Autodesk Inventor part; units mm, degrees
(part 3 of 3)
sketch "Sketch3" plane through (0, 0, 0) normal (0, -1, 0) x (1, 0, 0)
  line L0 (7.891, 22.7422) -> (7.891, -2.8235) construction
  line L1 (7.891, -2.8235) -> (4.151, -2.8235) construction
  line L2 (4.151, -2.8235) -> (4.151, 22.7422) construction
  line L3 (4.151, 22.7422) -> (7.891, 22.7422) construction
  line L4 (5.4758, -4.9863) -> (5.4758, -20.3165) construction
  line L5 (5.4758, -20.3165) -> (-4.0194, -20.3165) construction
  line L6 (-4.0194, -20.3165) -> (-4.0194, -4.9863) construction
  line L7 (-4.0194, -4.9863) -> (5.4758, -4.9863) construction
  line L8 (4.2338, 13.0137) -> (4.2338, 14.1137)
  line L9 (4.2338, 14.1137) -> (5.5167, 15.068)
  line L10 (5.5167, 15.068) -> (5.5167, 15.488)
  line L11 (5.5167, 15.488) -> (4.2338, 15.488)
  line L12 (4.2338, 15.488) -> (4.2338, 16.3851)
  line L13 (4.2338, 16.3851) -> (7.7338, 16.3851)
  line L14 (7.7338, 16.3851) -> (7.7338, 14.8708)
  spline S0 degree 2 poles (7.7338, 14.8708) (7.7338, 14.5594) (7.6624, 14.1137) (7.5453, 13.9194) knots 0 0 0 1 2 2 2
  spline S1 degree 2 poles (7.5453, 13.9194) (7.4281, 13.7194) (7.0538, 13.488) (6.771, 13.488) knots 0 0 0 1 2 2 2
  spline S2 degree 2 poles (6.771, 13.488) (6.3853, 13.488) (5.8938, 13.848) (5.7338, 14.1822) knots 0 0 0 1 2 2 2
  line L15 (5.7338, 14.1822) -> (4.2338, 13.0137)
  spline S3 degree 2 poles (6.6624, 14.4222) (6.7938, 14.4222) (6.9824, 14.5308) (7.0367, 14.6622) knots 0 0 0 1 2 2 2
  spline S4 degree 2 poles (7.0367, 14.6622) (7.0738, 14.7537) (7.091, 14.9994) (7.091, 15.1622) knots 0 0 0 1 2 2 2
  line L16 (7.091, 15.1622) -> (7.091, 15.488)
  line L17 (7.091, 15.488) -> (6.1481, 15.488)
  line L18 (6.1481, 15.488) -> (6.1481, 15.2108)
  spline S5 degree 2 poles (6.1481, 15.2108) (6.1481, 14.9937) (6.191, 14.7022) (6.2653, 14.6022) knots 0 0 0 1 2 2 2
  spline S6 degree 2 poles (6.2653, 14.6022) (6.3395, 14.508) (6.5138, 14.4222) (6.6624, 14.4222) knots 0 0 0 1 2 2 2
  spline S7 degree 2 poles (5.5538, 9.9651) (4.9024, 9.9651) (4.151, 10.7251) (4.151, 11.4108) knots 0 0 0 1 2 2 2
  spline S8 degree 2 poles (4.151, 11.4108) (4.151, 12.0994) (4.9024, 12.8594) (5.5538, 12.8594) knots 0 0 0 1 2 2 2
  spline S9 degree 2 poles (5.5538, 12.8594) (6.2081, 12.8594) (6.9567, 12.0937) (6.9567, 11.4108) knots 0 0 0 1 2 2 2
  spline S10 degree 2 poles (6.9567, 11.4108) (6.9567, 10.7194) (6.2053, 9.9651) (5.5538, 9.9651) knots 0 0 0 1 2 2 2
  spline S11 degree 2 poles (4.911, 11.008) (5.0138, 10.9251) (5.2967, 10.8422) (5.5481, 10.8422) knots 0 0 0 1 2 2 2
  spline S12 degree 2 poles (5.5481, 10.8422) (5.7795, 10.8422) (6.0938, 10.928) (6.1881, 11.0022) knots 0 0 0 1 2 2 2
  spline S13 degree 2 poles (6.1881, 11.0022) (6.2853, 11.0765) (6.3653, 11.2908) (6.3653, 11.4108) knots 0 0 0 1 2 2 2
  spline S14 degree 2 poles (6.3653, 11.4108) (6.3653, 11.5337) (6.2995, 11.7251) (6.1995, 11.8137) knots 0 0 0 1 2 2 2
  spline S15 degree 2 poles (6.1995, 11.8137) (6.1081, 11.8908) (5.791, 11.9822) (5.5481, 11.9822) knots 0 0 0 1 2 2 2
  spline S16 degree 2 poles (5.5481, 11.9822) (5.331, 11.9822) (5.0138, 11.9022) (4.9195, 11.8251) knots 0 0 0 1 2 2 2
  spline S17 degree 2 poles (4.9195, 11.8251) (4.8281, 11.748) (4.7424, 11.5394) (4.7424, 11.4051) knots 0 0 0 1 2 2 2
  spline S18 degree 2 poles (4.7424, 11.4051) (4.7424, 11.2908) (4.8195, 11.0794) (4.911, 11.008) knots 0 0 0 1 2 2 2
  spline S19 degree 2 poles (5.591, 6.6051) (4.9681, 6.6051) (4.1824, 7.2937) (4.1824, 7.808) knots 0 0 0 1 2 2 2
  spline S20 degree 2 poles (4.1824, 7.808) (4.1824, 8.028) (4.2767, 8.3594) (4.3653, 8.5108) knots 0 0 0 1 2 2 2
  line L19 (4.3653, 8.5108) -> (4.2338, 8.5451)
  line L20 (4.2338, 8.5451) -> (4.2338, 9.3594)
  line L21 (4.2338, 9.3594) -> (7.891, 9.3594)
  line L22 (7.891, 9.3594) -> (7.891, 8.5108)
  line L23 (7.891, 8.5108) -> (6.5967, 8.5108)
  spline S21 degree 2 poles (6.5967, 8.5108) (6.7538, 8.3165) (6.9453, 7.9108) (6.9453, 7.6451) knots 0 0 0 1 2 2 2
  spline S22 degree 2 poles (6.9453, 7.6451) (6.9453, 7.1451) (6.2253, 6.6051) (5.591, 6.6051) knots 0 0 0 1 2 2 2
  spline S23 degree 2 poles (5.571, 7.4765) (5.9224, 7.4765) (6.3024, 7.7165) (6.3024, 8.0222) knots 0 0 0 1 2 2 2
  spline S24 degree 2 poles (6.3024, 8.0222) (6.3024, 8.1422) (6.231, 8.3965) (6.1624, 8.5108) knots 0 0 0 1 2 2 2
  line L24 (6.1624, 8.5108) -> (4.8424, 8.5108)
  spline S25 degree 2 poles (4.8424, 8.5108) (4.8081, 8.4194) (4.7853, 8.2565) (4.7853, 8.1394) knots 0 0 0 1 2 2 2
  spline S26 degree 2 poles (4.7853, 8.1394) (4.7853, 7.8051) (5.1795, 7.4765) (5.571, 7.4765) knots 0 0 0 1 2 2 2
  spline S27 degree 2 poles (5.5538, 3.2937) (4.9024, 3.2937) (4.151, 4.0537) (4.151, 4.7394) knots 0 0 0 1 2 2 2
  spline S28 degree 2 poles (4.151, 4.7394) (4.151, 5.428) (4.9024, 6.188) (5.5538, 6.188) knots 0 0 0 1 2 2 2
  spline S29 degree 2 poles (5.5538, 6.188) (6.2081, 6.188) (6.9567, 5.4222) (6.9567, 4.7394) knots 0 0 0 1 2 2 2
  spline S30 degree 2 poles (6.9567, 4.7394) (6.9567, 4.048) (6.2053, 3.2937) (5.5538, 3.2937) knots 0 0 0 1 2 2 2
  spline S31 degree 2 poles (4.911, 4.3365) (5.0138, 4.2537) (5.2967, 4.1708) (5.5481, 4.1708) knots 0 0 0 1 2 2 2
  spline S32 degree 2 poles (5.5481, 4.1708) (5.7795, 4.1708) (6.0938, 4.2565) (6.1881, 4.3308) knots 0 0 0 1 2 2 2
  spline S33 degree 2 poles (6.1881, 4.3308) (6.2853, 4.4051) (6.3653, 4.6194) (6.3653, 4.7394) knots 0 0 0 1 2 2 2
  spline S34 degree 2 poles (6.3653, 4.7394) (6.3653, 4.8622) (6.2995, 5.0537) (6.1995, 5.1422) knots 0 0 0 1 2 2 2
  spline S35 degree 2 poles (6.1995, 5.1422) (6.1081, 5.2194) (5.791, 5.3108) (5.5481, 5.3108) knots 0 0 0 1 2 2 2
  spline S36 degree 2 poles (5.5481, 5.3108) (5.331, 5.3108) (5.0138, 5.2308) (4.9195, 5.1537) knots 0 0 0 1 2 2 2
  spline S37 degree 2 poles (4.9195, 5.1537) (4.8281, 5.0765) (4.7424, 4.868) (4.7424, 4.7337) knots 0 0 0 1 2 2 2
  spline S38 degree 2 poles (4.7424, 4.7337) (4.7424, 4.6194) (4.8195, 4.408) (4.911, 4.3365) knots 0 0 0 1 2 2 2
  spline S39 degree 2 poles (-0.5256, 12.428) (-0.7799, 12.428) (-1.1799, 12.6337) (-1.3113, 12.8108) knots 0 0 0 1 2 2 2
  spline S40 degree 2 poles (-1.3113, 12.8108) (-1.4656, 13.0194) (-1.5971, 13.5137) (-1.5971, 13.8965) knots 0 0 0 1 2 2 2
  line L25 (-1.5971, 13.8965) -> (-1.5971, 15.4251)
  line L26 (-1.5971, 15.4251) -> (1.9029, 15.4251)
  line L27 (1.9029, 15.4251) -> (1.9029, 14.0651)
  spline S41 degree 2 poles (1.9029, 14.0651) (1.9029, 13.6422) (1.8458, 13.2508) (1.7515, 13.0565) knots 0 0 0 1 2 2 2
  spline S42 degree 2 poles (1.7515, 13.0565) (1.6487, 12.8565) (1.3087, 12.6622) (1.0887, 12.6622) knots 0 0 0 1 2 2 2
  spline S43 degree 2 poles (1.0887, 12.6622) (0.8344, 12.6622) (0.4487, 12.9308) (0.3401, 13.1765) knots 0 0 0 1 2 2 2
  line L28 (0.3401, 13.1765) -> (0.3201, 13.1765)
  spline S44 degree 2 poles (0.3201, 13.1765) (0.2515, 12.8308) (-0.1742, 12.428) (-0.5256, 12.428) knots 0 0 0 1 2 2 2
  spline S45 degree 2 poles (-0.5113, 13.3651) (-0.3428, 13.3651) (-0.1628, 13.4937) (-0.1171, 13.6508) knots 0 0 0 1 2 2 2
  spline S46 degree 2 poles (-0.1171, 13.6508) (-0.0885, 13.7565) (-0.0828, 14.128) (-0.0828, 14.3308) knots 0 0 0 1 2 2 2
  line L29 (-0.0828, 14.3308) -> (-0.0828, 14.528)
  line L30 (-0.0828, 14.528) -> (-0.9542, 14.528)
  line L31 (-0.9542, 14.528) -> (-0.9542, 14.4622)
  spline S47 degree 2 poles (-0.9542, 14.4622) (-0.9542, 14.0794) (-0.9485, 13.7508) (-0.8913, 13.6137) knots 0 0 0 1 2 2 2
  spline S48 degree 2 poles (-0.8913, 13.6137) (-0.8313, 13.4708) (-0.6371, 13.3651) (-0.5113, 13.3651) knots 0 0 0 1 2 2 2
  spline S49 degree 2 poles (0.9115, 13.5851) (1.0001, 13.5851) (1.1744, 13.6737) (1.2144, 13.7822) knots 0 0 0 1 2 2 2
  spline S50 degree 2 poles (1.2144, 13.7822) (1.2544, 13.8822) (1.2601, 14.1765) (1.2601, 14.4422) knots 0 0 0 1 2 2 2
  line L32 (1.2601, 14.4422) -> (1.2601, 14.528)
  line L33 (1.2601, 14.528) -> (0.5201, 14.528)
  line L34 (0.5201, 14.528) -> (0.5201, 14.3851)
  spline S51 degree 2 poles (0.5201, 14.3851) (0.5201, 14.1708) (0.5344, 13.8708) (0.5744, 13.7822) knots 0 0 0 1 2 2 2
  spline S52 degree 2 poles (0.5744, 13.7822) (0.6287, 13.6594) (0.8001, 13.5851) (0.9115, 13.5851) knots 0 0 0 1 2 2 2
  line L35 (0.2372, 9.888) -> (0.2372, 9.9622)
  spline S53 degree 2 poles (0.2372, 9.9622) (0.2572, 10.0165) (0.2744, 10.2565) (0.2744, 10.3365) knots 0 0 0 1 2 2 2
  spline S54 degree 2 poles (0.2744, 10.3365) (0.2744, 10.5165) (0.2287, 10.7937) (0.1715, 10.9537) knots 0 0 0 1 2 2 2
  line L36 (0.1715, 10.9537) -> (-1.5971, 10.9537)
  line L37 (-1.5971, 10.9537) -> (-1.5971, 11.8022)
  line L38 (-1.5971, 11.8022) -> (1.0429, 11.8022)
  line L39 (1.0429, 11.8022) -> (1.0429, 10.9537)
  line L40 (1.0429, 10.9537) -> (0.6544, 10.9537)
  spline S55 degree 2 poles (0.6544, 10.9537) (0.8944, 10.6737) (1.0515, 10.2622) (1.0515, 10.088) knots 0 0 0 1 2 2 2
  spline S56 degree 2 poles (1.0515, 10.088) (1.0515, 10.0422) (1.0458, 9.9308) (1.0429, 9.888) knots 0 0 0 1 2 2 2
  line L41 (1.0429, 9.888) -> (0.2372, 9.888)
  line L42 (0.2372, 7.4937) -> (0.2372, 7.568)
  spline S57 degree 2 poles (0.2372, 7.568) (0.2572, 7.6222) (0.2744, 7.8622) (0.2744, 7.9422) knots 0 0 0 1 2 2 2
  spline S58 degree 2 poles (0.2744, 7.9422) (0.2744, 8.1222) (0.2287, 8.3994) (0.1715, 8.5594) knots 0 0 0 1 2 2 2
  line L43 (0.1715, 8.5594) -> (-1.5971, 8.5594)
  line L44 (-1.5971, 8.5594) -> (-1.5971, 9.408)
  line L45 (-1.5971, 9.408) -> (1.0429, 9.408)
  line L46 (1.0429, 9.408) -> (1.0429, 8.5594)
  line L47 (1.0429, 8.5594) -> (0.6544, 8.5594)
  spline S59 degree 2 poles (0.6544, 8.5594) (0.8944, 8.2794) (1.0515, 7.868) (1.0515, 7.6937) knots 0 0 0 1 2 2 2
  spline S60 degree 2 poles (1.0515, 7.6937) (1.0515, 7.648) (1.0458, 7.5365) (1.0429, 7.4937) knots 0 0 0 1 2 2 2
  line L48 (1.0429, 7.4937) -> (0.2372, 7.4937)
  line L49 (-1.5971, 4.448) -> (-1.5971, 5.2965)
  line L50 (-1.5971, 5.2965) -> (-1.3228, 5.2965)
  spline S61 degree 2 poles (-1.3228, 5.2965) (-1.4999, 5.5137) (-1.6713, 5.8937) (-1.6713, 6.1451) knots 0 0 0 1 2 2 2
  spline S62 degree 2 poles (-1.6713, 6.1451) (-1.6713, 6.6251) (-0.9285, 7.2022) (-0.2971, 7.2022) knots 0 0 0 1 2 2 2
  spline S63 degree 2 poles (-0.2971, 7.2022) (0.0372, 7.2022) (0.5572, 7.008) (0.7429, 6.8394) knots 0 0 0 1 2 2 2
  spline S64 degree 2 poles (0.7429, 6.8394) (0.9201, 6.6794) (1.1144, 6.2222) (1.1144, 5.9965) knots 0 0 0 1 2 2 2
  spline S65 degree 2 poles (1.1144, 5.9965) (1.1144, 5.7594) (1.0144, 5.4565) (0.9344, 5.2965) knots 0 0 0 1 2 2 2
  line L51 (0.9344, 5.2965) -> (2.0601, 5.2965)
  line L52 (2.0601, 5.2965) -> (2.0601, 4.448)
  line L53 (2.0601, 4.448) -> (-1.5971, 4.448)
  line L54 (-0.8713, 5.2965) -> (0.4258, 5.2965)
  spline S66 degree 2 poles (0.4258, 5.2965) (0.4629, 5.3851) (0.4972, 5.5822) (0.4972, 5.6651) knots 0 0 0 1 2 2 2
  spline S67 degree 2 poles (0.4972, 5.6651) (0.4972, 5.9965) (0.0801, 6.3308) (-0.2885, 6.3308) knots 0 0 0 1 2 2 2
  spline S68 degree 2 poles (-0.2885, 6.3308) (-0.6771, 6.3308) (-1.0285, 6.0622) (-1.0285, 5.768) knots 0 0 0 1 2 2 2
  spline S69 degree 2 poles (-1.0285, 5.768) (-1.0285, 5.6537) (-0.9428, 5.3937) (-0.8713, 5.2965) knots 0 0 0 1 2 2 2
  line L55 (-7.4279, 15.1337) -> (-7.4279, 16.0137)
  line L56 (-7.4279, 16.0137) -> (-6.5051, 16.0137)
  line L57 (-6.5051, 16.0137) -> (-6.5051, 15.1337)
  line L58 (-6.5051, 15.1337) -> (-7.4279, 15.1337)
  spline S70 degree 2 poles (-7.4994, 12.9308) (-7.4994, 13.2765) (-7.3336, 13.848) (-7.1622, 14.0594) knots 0 0 0 1 2 2 2
  spline S71 degree 2 poles (-7.1622, 14.0594) (-6.9908, 14.268) (-6.4708, 14.4994) (-6.1194, 14.4994) knots 0 0 0 1 2 2 2
  spline S72 degree 2 poles (-6.1194, 14.4994) (-5.7508, 14.4994) (-5.2136, 14.2537) (-5.0394, 14.0308) knots 0 0 0 1 2 2 2
  spline S73 degree 2 poles (-5.0394, 14.0308) (-4.8708, 13.8165) (-4.7165, 13.2594) (-4.7165, 12.9565) knots 0 0 0 1 2 2 2
  spline S74 degree 2 poles (-4.7165, 12.9565) (-4.7165, 12.688) (-4.8336, 12.2308) (-4.9279, 12.0337) knots 0 0 0 1 2 2 2
  line L59 (-4.9279, 12.0337) -> (-5.6508, 12.0337)
  line L60 (-5.6508, 12.0337) -> (-5.6508, 12.1537)
  spline S75 degree 2 poles (-5.6508, 12.1537) (-5.6079, 12.2022) (-5.4936, 12.3422) (-5.4394, 12.4422) knots 0 0 0 1 2 2 2
  spline S76 degree 2 poles (-5.4394, 12.4422) (-5.3879, 12.5394) (-5.3194, 12.768) (-5.3194, 12.9194) knots 0 0 0 1 2 2 2
  spline S77 degree 2 poles (-5.3194, 12.9194) (-5.3194, 13.2594) (-5.7508, 13.6222) (-6.1194, 13.6222) knots 0 0 0 1 2 2 2
  spline S78 degree 2 poles (-6.1194, 13.6222) (-6.5022, 13.6222) (-6.8965, 13.248) (-6.8965, 12.908) knots 0 0 0 1 2 2 2
  spline S79 degree 2 poles (-6.8965, 12.908) (-6.8965, 12.748) (-6.8222, 12.4908) (-6.7736, 12.408) knots 0 0 0 1 2 2 2
  spline S80 degree 2 poles (-6.7736, 12.408) (-6.7279, 12.328) (-6.6222, 12.2051) (-6.5736, 12.1537) knots 0 0 0 1 2 2 2
  line L61 (-6.5736, 12.1537) -> (-6.5736, 12.0337)
  line L62 (-6.5736, 12.0337) -> (-7.2936, 12.0337)
  spline S81 degree 2 poles (-7.2936, 12.0337) (-7.3879, 12.2337) (-7.4994, 12.668) (-7.4994, 12.9308) knots 0 0 0 1 2 2 2
  spline S82 degree 2 poles (-6.1079, 8.7737) (-6.7594, 8.7737) (-7.5108, 9.5337) (-7.5108, 10.2194) knots 0 0 0 1 2 2 2
  spline S83 degree 2 poles (-7.5108, 10.2194) (-7.5108, 10.908) (-6.7594, 11.668) (-6.1079, 11.668) knots 0 0 0 1 2 2 2
  spline S84 degree 2 poles (-6.1079, 11.668) (-5.4536, 11.668) (-4.7051, 10.9022) (-4.7051, 10.2194) knots 0 0 0 1 2 2 2
  spline S85 degree 2 poles (-4.7051, 10.2194) (-4.7051, 9.528) (-5.4565, 8.7737) (-6.1079, 8.7737) knots 0 0 0 1 2 2 2
  spline S86 degree 2 poles (-6.7508, 9.8165) (-6.6479, 9.7337) (-6.3651, 9.6508) (-6.1136, 9.6508) knots 0 0 0 1 2 2 2
  spline S87 degree 2 poles (-6.1136, 9.6508) (-5.8822, 9.6508) (-5.5679, 9.7365) (-5.4736, 9.8108) knots 0 0 0 1 2 2 2
  spline S88 degree 2 poles (-5.4736, 9.8108) (-5.3765, 9.8851) (-5.2965, 10.0994) (-5.2965, 10.2194) knots 0 0 0 1 2 2 2
  spline S89 degree 2 poles (-5.2965, 10.2194) (-5.2965, 10.3422) (-5.3622, 10.5337) (-5.4622, 10.6222) knots 0 0 0 1 2 2 2
  spline S90 degree 2 poles (-5.4622, 10.6222) (-5.5536, 10.6994) (-5.8708, 10.7908) (-6.1136, 10.7908) knots 0 0 0 1 2 2 2
  spline S91 degree 2 poles (-6.1136, 10.7908) (-6.3308, 10.7908) (-6.6479, 10.7108) (-6.7422, 10.6337) knots 0 0 0 1 2 2 2
  spline S92 degree 2 poles (-6.7422, 10.6337) (-6.8336, 10.5565) (-6.9194, 10.348) (-6.9194, 10.2137) knots 0 0 0 1 2 2 2
  spline S93 degree 2 poles (-6.9194, 10.2137) (-6.9194, 10.0994) (-6.8422, 9.888) (-6.7508, 9.8165) knots 0 0 0 1 2 2 2
  line L63 (-5.5565, 5.5908) -> (-7.4279, 5.5908)
  line L64 (-7.4279, 5.5908) -> (-7.4279, 6.4394)
  line L65 (-7.4279, 6.4394) -> (-6.1079, 6.4394)
  spline S94 degree 2 poles (-6.1079, 6.4394) (-5.9165, 6.4394) (-5.6451, 6.4594) (-5.5622, 6.4994) knots 0 0 0 1 2 2 2
  spline S95 degree 2 poles (-5.5622, 6.4994) (-5.4765, 6.5422) (-5.3994, 6.7137) (-5.3994, 6.868) knots 0 0 0 1 2 2 2
  spline S96 degree 2 poles (-5.3994, 6.868) (-5.3994, 6.9937) (-5.4994, 7.228) (-5.5565, 7.3222) knots 0 0 0 1 2 2 2
  line L66 (-5.5565, 7.3222) -> (-7.4279, 7.3222)
  line L67 (-7.4279, 7.3222) -> (-7.4279, 8.1708)
  line L68 (-7.4279, 8.1708) -> (-4.7879, 8.1708)
  line L69 (-4.7879, 8.1708) -> (-4.7879, 7.3222)
  line L70 (-4.7879, 7.3222) -> (-5.0794, 7.3222)
  spline S97 degree 2 poles (-5.0794, 7.3222) (-4.9079, 7.1051) (-4.7165, 6.7051) (-4.7165, 6.4622) knots 0 0 0 1 2 2 2
  spline S98 degree 2 poles (-4.7165, 6.4622) (-4.7165, 6.2022) (-4.9479, 5.8051) (-5.1736, 5.6908) knots 0 0 0 1 2 2 2
  spline S99 degree 2 poles (-5.1736, 5.6908) (-4.9622, 5.4394) (-4.7165, 4.9594) (-4.7165, 4.7308) knots 0 0 0 1 2 2 2
  spline S100 degree 2 poles (-4.7165, 4.7308) (-4.7165, 4.3022) (-5.2279, 3.8594) (-5.7108, 3.8594) knots 0 0 0 1 2 2 2
  line L71 (-5.7108, 3.8594) -> (-7.4279, 3.8594)
  line L72 (-7.4279, 3.8594) -> (-7.4279, 4.708)
  line L73 (-7.4279, 4.708) -> (-6.1079, 4.708)
  spline S101 degree 2 poles (-6.1079, 4.708) (-5.9136, 4.708) (-5.6451, 4.7251) (-5.5622, 4.768) knots 0 0 0 1 2 2 2
  spline S102 degree 2 poles (-5.5622, 4.768) (-5.4765, 4.808) (-5.3994, 4.9794) (-5.3994, 5.1365) knots 0 0 0 1 2 2 2
  spline S103 degree 2 poles (-5.3994, 5.1365) (-5.3994, 5.2422) (-5.4708, 5.4451) (-5.5565, 5.5908) knots 0 0 0 1 2 2 2
  spline S104 degree 2 poles (1.3452, -5.9852) (1.0774, -5.995) (0.8423, -6.2628) (0.8423, -6.5893) knots 0 0 0 1 2 2 2
  spline S105 degree 2 poles (0.8423, -6.5893) (0.8423, -6.7003) (0.9174, -7.0008) (0.9468, -7.0595) knots 0 0 0 1 2 2 2
  line L74 (0.9468, -7.0595) -> (0.9468, -7.1608)
  line L75 (0.9468, -7.1608) -> (0.2415, -7.1608)
  spline S106 degree 2 poles (0.2415, -7.1608) (0.2056, -7.0106) (0.1534, -6.6579) (0.1534, -6.2954) knots 0 0 0 1 2 2 2
  spline S107 degree 2 poles (0.1534, -6.2954) (0.1534, -5.9754) (0.3134, -5.502) (0.457, -5.342) knots 0 0 0 1 2 2 2
  spline S108 degree 2 poles (0.457, -5.342) (0.6007, -5.1885) (0.986, -5.0318) (1.2244, -5.0187) knots 0 0 0 1 2 2 2
  spline S109 degree 2 poles (1.2244, -5.0187) (1.2766, -4.124) (2.3738, -3.1216) (3.2946, -3.1216) knots 0 0 0 1 2 2 2
  spline S110 degree 2 poles (3.2946, -3.1216) (4.2611, -3.1216) (5.3811, -4.2154) (5.3811, -5.182) knots 0 0 0 1 2 2 2
  spline S111 degree 2 poles (5.3811, -5.182) (5.3811, -6.142) (4.2611, -7.2424) (3.2946, -7.2424) knots 0 0 0 1 2 2 2
  spline S112 degree 2 poles (3.2946, -7.2424) (2.5827, -7.2424) (1.5509, -6.5991) (1.3452, -5.9852) knots 0 0 0 1 2 2 2
  spline S113 degree 2 poles (2.2823, -5.8775) (2.4652, -6.0277) (2.9648, -6.1714) (3.2979, -6.1714) knots 0 0 0 1 2 2 2
  spline S114 degree 2 poles (3.2979, -6.1714) (3.6603, -6.1714) (4.1632, -6.0048) (4.3199, -5.871) knots 0 0 0 1 2 2 2
  spline S115 degree 2 poles (4.3199, -5.871) (4.4832, -5.7338) (4.6268, -5.3779) (4.6268, -5.182) knots 0 0 0 1 2 2 2
  spline S116 degree 2 poles (4.6268, -5.182) (4.6268, -4.9861) (4.4864, -4.6399) (4.3264, -4.4963) knots 0 0 0 1 2 2 2
  spline S117 degree 2 poles (4.3264, -4.4963) (4.1762, -4.3624) (3.6472, -4.1926) (3.2979, -4.1926) knots 0 0 0 1 2 2 2
  spline S118 degree 2 poles (3.2979, -4.1926) (2.9387, -4.1926) (2.4358, -4.3559) (2.2791, -4.4897) knots 0 0 0 1 2 2 2
  spline S119 degree 2 poles (2.2791, -4.4897) (2.1191, -4.6236) (1.9689, -4.9861) (1.9689, -5.182) knots 0 0 0 1 2 2 2
  spline S120 degree 2 poles (1.9689, -5.182) (1.9689, -5.3812) (2.1223, -5.7403) (2.2823, -5.8775) knots 0 0 0 1 2 2 2
  line L76 (1.2962, -10.9812) -> (1.2962, -10.0114)
  line L77 (1.2962, -10.0114) -> (1.6293, -10.0114)
  spline S121 degree 2 poles (1.6293, -10.0114) (1.4236, -9.7436) (1.2113, -9.2963) (1.2113, -8.9893) knots 0 0 0 1 2 2 2
  spline S122 degree 2 poles (1.2113, -8.9893) (1.2113, -8.4897) (1.786, -7.951) (2.3476, -7.951) knots 0 0 0 1 2 2 2
  line L78 (2.3476, -7.951) -> (4.3134, -7.951)
  line L79 (4.3134, -7.951) -> (4.3134, -8.9208)
  line L80 (4.3134, -8.9208) -> (2.8146, -8.9208)
  spline S123 degree 2 poles (2.8146, -8.9208) (2.586, -8.9208) (2.2823, -8.9501) (2.1844, -9.0057) knots 0 0 0 1 2 2 2
  spline S124 degree 2 poles (2.1844, -9.0057) (2.0832, -9.0546) (1.9917, -9.2603) (1.9917, -9.4465) knots 0 0 0 1 2 2 2
  spline S125 degree 2 poles (1.9917, -9.4465) (1.9917, -9.5706) (2.0832, -9.871) (2.1713, -10.0114) knots 0 0 0 1 2 2 2
  line L81 (2.1713, -10.0114) -> (4.3134, -10.0114)
  line L82 (4.3134, -10.0114) -> (4.3134, -10.9812)
  line L83 (4.3134, -10.9812) -> (1.2962, -10.9812)
  line L84 (1.2962, -12.8652) -> (1.2962, -11.8954)
  line L85 (1.2962, -11.8954) -> (4.3134, -11.8954)
  line L86 (4.3134, -11.8954) -> (4.3134, -12.8652)
  line L87 (4.3134, -12.8652) -> (1.2962, -12.8652)
  line L88 (4.7411, -12.8914) -> (4.7411, -11.8693)
  line L89 (4.7411, -11.8693) -> (5.4758, -11.8693)
  line L90 (5.4758, -11.8693) -> (5.4758, -12.8914)
  line L91 (5.4758, -12.8914) -> (4.7411, -12.8914)
  spline S126 degree 2 poles (1.2146, -15.3469) (1.2146, -14.9518) (1.404, -14.2987) (1.5999, -14.0571) knots 0 0 0 1 2 2 2
  spline S127 degree 2 poles (1.5999, -14.0571) (1.7958, -13.8187) (2.3901, -13.5542) (2.7917, -13.5542) knots 0 0 0 1 2 2 2
  spline S128 degree 2 poles (2.7917, -13.5542) (3.213, -13.5542) (3.8268, -13.835) (4.026, -14.0897) knots 0 0 0 1 2 2 2
  spline S129 degree 2 poles (4.026, -14.0897) (4.2187, -14.3346) (4.395, -14.9714) (4.395, -15.3175) knots 0 0 0 1 2 2 2
  spline S130 degree 2 poles (4.395, -15.3175) (4.395, -15.6244) (4.2611, -16.1469) (4.1534, -16.3722) knots 0 0 0 1 2 2 2
  line L92 (4.1534, -16.3722) -> (3.3272, -16.3722)
  line L93 (3.3272, -16.3722) -> (3.3272, -16.235)
  spline S131 degree 2 poles (3.3272, -16.235) (3.3762, -16.1795) (3.5068, -16.0195) (3.5689, -15.9052) knots 0 0 0 1 2 2 2
  spline S132 degree 2 poles (3.5689, -15.9052) (3.6276, -15.7942) (3.706, -15.533) (3.706, -15.3599) knots 0 0 0 1 2 2 2
  spline S133 degree 2 poles (3.706, -15.3599) (3.706, -14.9714) (3.213, -14.5567) (2.7917, -14.5567) knots 0 0 0 1 2 2 2
  spline S134 degree 2 poles (2.7917, -14.5567) (2.3542, -14.5567) (1.9036, -14.9844) (1.9036, -15.373) knots 0 0 0 1 2 2 2
  spline S135 degree 2 poles (1.9036, -15.373) (1.9036, -15.5559) (1.9885, -15.8497) (2.044, -15.9444) knots 0 0 0 1 2 2 2
  spline S136 degree 2 poles (2.044, -15.9444) (2.0962, -16.0359) (2.217, -16.1763) (2.2725, -16.235) knots 0 0 0 1 2 2 2
  line L94 (2.2725, -16.235) -> (2.2725, -16.3722)
  line L95 (2.2725, -16.3722) -> (1.4497, -16.3722)
  spline S137 degree 2 poles (1.4497, -16.3722) (1.3419, -16.1436) (1.2146, -15.6473) (1.2146, -15.3469) knots 0 0 0 1 2 2 2
  line L96 (1.2962, -20.2122) -> (1.2962, -19.0889)
  line L97 (1.2962, -19.0889) -> (2.6089, -18.2432)
  line L98 (2.6089, -18.2432) -> (2.2856, -17.982)
  line L99 (2.2856, -17.982) -> (1.2962, -17.982)
  line L100 (1.2962, -17.982) -> (1.2962, -17.0122)
  line L101 (1.2962, -17.0122) -> (5.4758, -17.0122)
  line L102 (5.4758, -17.0122) -> (5.4758, -17.982)
  line L103 (5.4758, -17.982) -> (2.9876, -17.982)
  line L104 (2.9876, -17.982) -> (4.3134, -19.0171)
  line L105 (4.3134, -19.0171) -> (4.3134, -20.1338)
  line L106 (4.3134, -20.1338) -> (3.0138, -19.053)
  line L107 (3.0138, -19.053) -> (1.2962, -20.2122)
  line L108 (5.2962, -21.9134) -> (2.4489, -21.7893)
  line L109 (2.4489, -21.7893) -> (2.4489, -20.9142)
  line L110 (2.4489, -20.9142) -> (5.2962, -20.7901)
  line L111 (5.2962, -20.7901) -> (5.2962, -21.9134)
  line L112 (1.2962, -21.8938) -> (1.2962, -20.8097)
  line L113 (1.2962, -20.8097) -> (2.0048, -20.8097)
  line L114 (2.0048, -20.8097) -> (2.0048, -21.8938)
  line L115 (2.0048, -21.8938) -> (1.2962, -21.8938)
  line L116 (-1.3676, -8.9289) -> (-5.3676, -7.4693)
  line L117 (-5.3676, -7.4693) -> (-5.3676, -6.3167)
  line L118 (-5.3676, -6.3167) -> (-1.3676, -4.8571)
  line L119 (-1.3676, -4.8571) -> (-1.3676, -5.9379)
  line L120 (-1.3676, -5.9379) -> (-4.1758, -6.9044)
  line L121 (-4.1758, -6.9044) -> (-1.3676, -7.871)
  line L122 (-1.3676, -7.871) -> (-1.3676, -8.9289)
  line L123 (-5.3676, -12.3836) -> (-5.3676, -11.4138)
  line L124 (-5.3676, -11.4138) -> (-5.0542, -11.4138)
  spline S138 degree 2 poles (-5.0542, -11.4138) (-5.2566, -11.1657) (-5.4525, -10.7314) (-5.4525, -10.444) knots 0 0 0 1 2 2 2
  spline S139 degree 2 poles (-5.4525, -10.444) (-5.4525, -9.8954) (-4.6036, -9.2359) (-3.8819, -9.2359) knots 0 0 0 1 2 2 2
  spline S140 degree 2 poles (-3.8819, -9.2359) (-3.4999, -9.2359) (-2.9056, -9.4579) (-2.6934, -9.6506) knots 0 0 0 1 2 2 2
  spline S141 degree 2 poles (-2.6934, -9.6506) (-2.4909, -9.8334) (-2.2689, -10.3559) (-2.2689, -10.6138) knots 0 0 0 1 2 2 2
  spline S142 degree 2 poles (-2.2689, -10.6138) (-2.2689, -10.8848) (-2.3832, -11.231) (-2.4746, -11.4138) knots 0 0 0 1 2 2 2
  line L125 (-2.4746, -11.4138) -> (-1.1881, -11.4138)
  line L126 (-1.1881, -11.4138) -> (-1.1881, -12.3836)
  line L127 (-1.1881, -12.3836) -> (-5.3676, -12.3836)
  line L128 (-4.5383, -11.4138) -> (-3.0558, -11.4138)
  spline S143 degree 2 poles (-3.0558, -11.4138) (-3.0134, -11.3126) (-2.9742, -11.0873) (-2.9742, -10.9926) knots 0 0 0 1 2 2 2
  spline S144 degree 2 poles (-2.9742, -10.9926) (-2.9742, -10.6138) (-3.4509, -10.2318) (-3.8721, -10.2318) knots 0 0 0 1 2 2 2
  spline S145 degree 2 poles (-3.8721, -10.2318) (-4.3162, -10.2318) (-4.7178, -10.5387) (-4.7178, -10.875) knots 0 0 0 1 2 2 2
  spline S146 degree 2 poles (-4.7178, -10.875) (-4.7178, -11.0057) (-4.6199, -11.3028) (-4.5383, -11.4138) knots 0 0 0 1 2 2 2
  line L129 (-5.3676, -14.2677) -> (-5.3676, -13.2979)
  line L130 (-5.3676, -13.2979) -> (-2.3505, -13.2979)
  line L131 (-2.3505, -13.2979) -> (-2.3505, -14.2677)
  line L132 (-2.3505, -14.2677) -> (-5.3676, -14.2677)
  line L133 (-1.9227, -14.2938) -> (-1.9227, -13.2718)
  line L134 (-1.9227, -13.2718) -> (-1.1881, -13.2718)
  line L135 (-1.1881, -13.2718) -> (-1.1881, -14.2938)
  line L136 (-1.1881, -14.2938) -> (-1.9227, -14.2938)
  line L137 (-2.3505, -18.2154) -> (-5.3676, -17.053)
  line L138 (-5.3676, -17.053) -> (-5.3676, -15.9591)
  line L139 (-5.3676, -15.9591) -> (-2.3505, -14.8032)
  line L140 (-2.3505, -14.8032) -> (-2.3505, -15.8252)
  line L141 (-2.3505, -15.8252) -> (-4.4272, -16.524)
  line L142 (-4.4272, -16.524) -> (-2.3505, -17.2163)
  line L143 (-2.3505, -17.2163) -> (-2.3505, -18.2154)
  line L144 (-1.3676, -19.9657) -> (-4.215, -19.8416)
  line L145 (-4.215, -19.8416) -> (-4.215, -18.9665)
  line L146 (-4.215, -18.9665) -> (-1.3676, -18.8424)
  line L147 (-1.3676, -18.8424) -> (-1.3676, -19.9657)
  line L148 (-5.3676, -19.9461) -> (-5.3676, -18.862)
  line L149 (-5.3676, -18.862) -> (-4.6591, -18.862)
  line L150 (-4.6591, -18.862) -> (-4.6591, -19.9461)
  line L151 (-4.6591, -19.9461) -> (-5.3676, -19.9461)
  point P0 (0, 0)
  constraints: 4 other
emboss "Emboss1" sketch "Sketch3" operation cut depth 0.54 direction (0, 1, 0)
body "Solid1"
